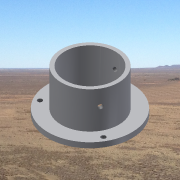
# Autodesk Inventor part: 2f1col
Saved by Autodesk Inventor 2013 SP2 (Build 170200200, 200)
## iProperties
Created: 2013-12-04
Part Number: 2f1col
Material: Aluminum 6061
Document SubType Name: Modeling
Designer: Dave
Mass: 197.234 g
Surface Area: 321.611 cm^2
Volume: 72.7802 cm^3
Density: 2.71 g/cm^3
Author: Dave
Autodesk Inventor part; units mm, degrees
ref_plane "YZ Plane" through (0, 0, 0) normal (1, 0, 0) x (0, 1, 0)
ref_plane "XZ Plane" through (0, 0, 0) normal (0, 1, 0) x (-1, 0, 0)
ref_plane "XY Plane" through (0, 0, 0) normal (0, 0, 1) x (1, 0, 0)
sketch "Sketch1" plane through (0, 0, 0) normal (0, 1, 0) x (-1, 0, 0)
  circle A0 centre (0, 0) radius 50.8
  dimension "d0" = 101.6
  constraints: 1 centre point, 1 coincident
  measures "d0" diameter of A0
extrude "Extrusion1" add sketch "Sketch1" along normal blind 50.8
sketch "Sketch2" plane through (0, 50.8, 0) normal (0, 1, 0) x (1, 0, 0)
  circle A0 centre (0, 0) radius 50.8 projected
  circle A1 centre (0, 0) radius 30.48
  dimension "d4" = 60.96
  constraints: 1 centre point, 1 coincident
  measures "d4" diameter of A1
extrude "Extrusion2" cut sketch "Sketch2" against normal blind 101.6 contours A1
sketch "Sketch3" plane through (0, 50.8, 0) normal (0, 1, 0) x (1, 0, 0)
  circle A0 centre (0, 0) radius 30.48 projected
  circle A1 centre (0, 0) radius 50.8 projected
  circle A2 centre (0, 0) radius 34.925
  dimension "d9" = 4.445
  constraints: 1 centre point
  measures "d9" radial gap between concentric circles of A0 A2
extrude "Extrusion3" cut sketch "Sketch3" against normal blind 44.45 contours A1
sketch "Sketch4" plane through (0, 50.8, 0) normal (0, 1, 0) x (1, 0, 0)
  circle A0 centre (0, 0) radius 34.925 projected
  circle A1 centre (0, 0) radius 30.48 projected
  point P0 (0, 34.925)
  constraints: 1 vertical alignment, 1 other
ref_plane "Work Plane1" through (0, 50.8, -34.925) normal (0, 0, -1) x (-1, 0, 0)
sketch "Sketch5" plane through (0, 50.8, -34.925) normal (0, 0, -1) x (-1, 0, 0)
  circle A0 centre (0, -19.05) radius 2.54
  line L0 (34.925, 0) -> (-34.925, 0) projected
  point P0 (0, -50.8)
  dimension "d12" = 19.05
  dimension "d13" = 5.08
  constraints: 1 centre point
  measures "d12" distance from line of A0.centre L0
  measures "d13" diameter of A0
hole "Hole1" at (0, 31.75, -34.925) direction (0, 0, 1) diameter 5.4864 depth 25.4 tip angle 118 thread size "1/4-32 UNEF" class "2B" standard "ANSI Unified Screw Threads"
pattern_circular "Circular Pattern1" count 3 over 360 about axis through (0, 50.8, 0) along (0, -1, 0) of "Hole1"
sketch "Sketch6" plane through (0, 6.35, 0) normal (0, 1, 0) x (1, 0, 0)
  circle A0 centre (0, 0) radius 34.925 projected
  circle A1 centre (0, 44.45) radius 2.2451
  dimension "d24" = 44.45
  constraints: 1 centre point
  measures "d24" distance of A0.centre A1.centre
hole "Hole2" at (0, 6.35, -44.45) direction (0, -1, 0) diameter 5.4864 depth 25.4 tip angle 118 thread size "1/4-32 UNEF" class "2B" standard "ANSI Unified Screw Threads"
pattern_circular "Circular Pattern2" count 3 over 360 about axis through (0, 0, 0) along (0, 1, 0) of "Hole2"
body "Solid1"
